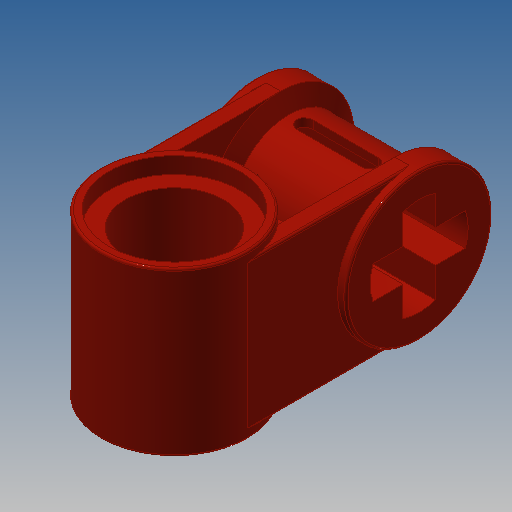
# Autodesk Inventor part: 6536-Red
Saved by Autodesk Inventor 2022.2 (Build 262287000, 287)
## iProperties
Created: 2014-07-19
Part Number: 6536-Red
Material: ABS Plastic
Document SubType Name: Modeling
Designer: D. Kohfeld
Mass: 0.381818 g
Surface Area: 7.9954 cm^2
Volume: 0.360206 cm^3
Density: 1.06 g/cm^3
Appearance: Red
Author: D. Kohfeld
Autodesk Inventor part; units mm, degrees
ref_plane "YZ Plane" through (0, 0, 0) normal (1, 0, 0) x (0, 1, 0)
ref_plane "XZ Plane" through (0, 0, 0) normal (0, 1, 0) x (-1, 0, 0)
sketch "Sketch2" plane through (0, 0, 0) normal (0, 1, 0) x (-1, 0, 0)
  circle A0 centre (0, 0) radius 3.6
  circle A1 centre (0, 0) radius 2.4
  line L0 (-3.6, -8) -> (3.6, -8)
  line L1 (-4, -8) -> (-4, -11.6)
  line L2 (-4, -11.6) -> (-2.8, -11.6)
  line L3 (-2.8, -11.6) -> (-2.4, -10.8)
  line L4 (-2.4, -10.8) -> (2.4, -10.8)
  line L5 (2.4, -10.8) -> (2.8, -11.6)
  line L6 (2.8, -11.6) -> (4, -11.6)
  line L7 (4, -11.6) -> (4, -8)
  line L8 (4, -8) -> (-4, -8)
  line L9 (3.6, -8) -> (3.6, 0)
  line L10 (-3.6, -8) -> (-3.6, 0)
  line L11 (-1.6, -7.6) -> (1.6, -7.6)
  arc A2 (1.6, -8.4) -> (1.6, -7.6) centre (1.6, -8) ccw
  line L12 (1.6, -8.4) -> (-1.6, -8.4)
  arc A3 (-1.6, -7.6) -> (-1.6, -8.4) centre (-1.6, -8) ccw
  point P0 (0, -8)
  point P1 (0, -7.6)
  dimension "d0" = 7.2
  dimension "d1" = 4.8
  dimension "d2" = 8
  dimension "d13" = 7.2
  dimension "d14" = 1.2
  dimension "d15" = 8
  dimension "d16" = 5.6
  dimension "d17" = 1.6
  dimension "d18" = 0.8
  dimension "d19" = 4
  constraints: 26 end point, 6 point on circle, 6 tangent, 4 centre point, 4 parallel, 3 equal length, 3 midpoint, 3 perpendicular, 2 coincident, 2 vertical, 1 collinear, 1 horizontal, 1 horizontal alignment, 1 vertical alignment
  measures "d0" diameter of A0
  measures "d1" diameter of A1
  measures "d2" distance from line of L0 A0.centre
  measures "d13" diameter of L2 L0
  measures "d14" distance from line of L2.end L1
  measures "d15" distance between parallel lines of L7 L1
  measures "d16" diameter of L4 L0
  measures "d17" distance from line of L3.end L1
  measures "d18" distance between parallel lines of L12 L11
sketch "Sketch2 outline for Extrusion1" plane through (0, 0, 0) normal (0, 1, 0) x (-1, 0, 0)
  circle A0 centre (0, 0) radius 3.6
  circle A1 centre (0, 0) radius 2.4
extrude "Extrusion1" add sketch "Sketch2 outline for Extrusion1" along normal mid plane 8
sketch "Sketch4" plane through (0, 4, 0) normal (0, 1, 0) x (1, 0, 0)
  circle A0 centre (0, 0) radius 2.4 projected
  circle A1 centre (0, 0) radius 3.6 projected
  circle A2 centre (0, 0) radius 3.2
  dimension "d10" = 6.4
  constraints: 1 centre point, 1 coincident
  measures "d10" diameter of A2
sketch "Sketch4 outline for Extrusion3" plane through (0, 4, 0) normal (0, 1, 0) x (1, 0, 0)
  circle A0 centre (0, 0) radius 3.2
  circle A1 centre (0, 0) radius 2.4
extrude "Extrusion3" cut sketch "Sketch4 outline for Extrusion3" against normal blind 0.8
mirror "Mirror1" about plane through (0, 0, 0) normal (0, 1, 0) of "Extrusion3"
ref_plane "Work Plane1" through (3.6, 0, -8) normal (0, 0, -1) x (-1, 0, 0)
sketch "Sketch3" plane through (3.6, 0, -8) normal (0, 0, -1) x (-1, 0, 0)
  line L0 (0, -4) -> (0, 4) projected
  line L1 (7.2, -4) -> (7.2, 4) projected
  line L2 (0, 3.6) -> (0.8, 3.6)
  line L3 (0.8, 3.6) -> (0.8, -3.6)
  line L4 (0.8, -3.6) -> (0, -3.6)
  line L5 (0, -3.6) -> (0, 3.6)
  line L6 (7.2, 3.6) -> (6.4, 3.6)
  line L7 (6.4, 3.6) -> (6.4, -3.6)
  line L8 (6.4, -3.6) -> (7.2, -3.6)
  line L9 (7.2, -3.6) -> (7.2, 3.6)
  point P0 (3.6, 0)
  point P1 (0, 0)
  point P2 (7.2, 0)
  dimension "d6" = 7.2
  dimension "d7" = 0.8
  constraints: 16 end point, 4 midpoint, 4 parallel, 2 equal length, 2 horizontal, 2 perpendicular, 2 point on line
  measures "d6" distance between parallel lines of L4 L2
  measures "d7" distance between parallel lines of L0 L3
sketch "Sketch3 outline for Extrusion2" plane through (3.6, 0, -8) normal (0, 0, -1) x (-1, 0, 0)
  line L0 (0.8, 3.6) -> (0, 3.6)
  line L1 (0, 3.6) -> (0, -3.6)
  line L2 (0, -3.6) -> (0.8, -3.6)
  line L3 (0.8, -3.6) -> (0.8, 3.6)
  line L4 (7.2, -3.6) -> (7.2, 3.6)
  line L5 (7.2, 3.6) -> (6.4, 3.6)
  line L6 (6.4, 3.6) -> (6.4, -3.6)
  line L7 (6.4, -3.6) -> (7.2, -3.6)
extrude "Extrusion2" add sketch "Sketch3 outline for Extrusion2" against normal up to next
sketch "Sketch2 outline for Revolution1" plane through (0, 0, 0) normal (0, 1, 0) x (-1, 0, 0)
  line L0 (-4, -11.6) -> (-4, -8)
  line L1 (-4, -8) -> (4, -8)
  line L2 (4, -8) -> (4, -11.6)
  line L3 (4, -11.6) -> (2.8, -11.6)
  line L4 (2.8, -11.6) -> (2.4, -10.8)
  line L5 (2.4, -10.8) -> (-2.4, -10.8)
  line L6 (-2.4, -10.8) -> (-2.8, -11.6)
  line L7 (-2.8, -11.6) -> (-4, -11.6)
revolve "Revolution1" add sketch "Sketch2 outline for Revolution1" angle 360 about axis through (-4, 0, -8) along (1, 0, 0)
sketch "Sketch2 outline for Extrusion4" plane through (0, 0, 0) normal (0, 1, 0) x (-1, 0, 0)
  line L0 (-3.6, 0) -> (-3.6, -8)
  arc A0 (3.6, 0) -> (-3.6, 0) centre (0, 0) cw
  line L1 (3.6, -8) -> (3.6, 0)
  line L2 (0, -8) -> (3.6, -8)
  line L3 (-3.6, -8) -> (0, -8)
extrude "Extrusion4" add sketch "Sketch2 outline for Extrusion4" along normal mid plane 1.6
sketch "Sketch2 outline for Extrusion5" plane through (0, 0, 0) normal (0, 1, 0) x (-1, 0, 0)
  line L0 (-1.6, -7.6) -> (1.6, -7.6)
  arc A0 (1.6, -7.6) -> (1.6, -8.4) centre (1.6, -8) cw
  line L1 (1.6, -8.4) -> (-1.6, -8.4)
  arc A1 (-1.6, -8.4) -> (-1.6, -7.6) centre (-1.6, -8) cw
extrude "Extrusion5" cut sketch "Sketch2 outline for Extrusion5" along normal through all both and the other way through all
sketch "Sketch5" plane through (4, 0, -8) normal (1, 0, 0) x (0, 0, -1)
  circle A0 centre (0, 0) radius 3.6
  circle A1 centre (0, 0) radius 2.4 construction
  line L0 (-0.8, 2.262742) -> (-0.8, 0.8)
  line L1 (-0.8, 0.8) -> (-2.262742, 0.8)
  line L2 (-2.262742, -0.8) -> (-0.8, -0.8)
  line L3 (-0.8, -0.8) -> (-0.8, -2.262742)
  line L4 (0.8, -2.262742) -> (0.8, -0.8)
  line L5 (0.8, -0.8) -> (2.262742, -0.8)
  line L6 (2.262742, 0.8) -> (0.8, 0.8)
  line L7 (0.8, 0.8) -> (0.8, 2.262742)
  arc A2 (0.8, 2.262742) -> (-0.8, 2.262742) centre (0, 0) ccw
  arc A3 (-2.262742, 0.8) -> (-2.262742, -0.8) centre (0, 0) ccw
  arc A4 (-0.8, -2.262742) -> (0.8, -2.262742) centre (0, 0) ccw
  arc A5 (2.262742, -0.8) -> (2.262742, 0.8) centre (0, 0) ccw
  point P0 (-8, 0)
  dimension "d25" = 4.8
  dimension "d26" = 1.6
  constraints: 16 end point, 8 point on circle, 7 equal length, 4 centre point, 4 perpendicular, 3 parallel, 1 coincident, 1 vertical, 14 other
  measures "d26" distance between parallel lines of L7 L0
sketch "Sketch5 outline for Extrusion6" plane through (4, 0, -8) normal (1, 0, 0) x (0, 0, -1)
  arc A0 (0.8, 2.262742) -> (-0.8, 2.262742) centre (0, 0) ccw
  line L0 (0.8, 0.8) -> (0.8, 2.262742)
  line L1 (2.262742, 0.8) -> (0.8, 0.8)
  arc A1 (2.262742, -0.8) -> (2.262742, 0.8) centre (0, 0) ccw
  line L2 (0.8, -0.8) -> (2.262742, -0.8)
  line L3 (0.8, -2.262742) -> (0.8, -0.8)
  arc A2 (-0.8, -2.262742) -> (0.8, -2.262742) centre (0, 0) ccw
  line L4 (-0.8, -0.8) -> (-0.8, -2.262742)
  line L5 (-2.262742, -0.8) -> (-0.8, -0.8)
  arc A3 (-2.262742, 0.8) -> (-2.262742, -0.8) centre (0, 0) ccw
  line L6 (-0.8, 0.8) -> (-2.262742, 0.8)
  line L7 (-0.8, 2.262742) -> (-0.8, 0.8)
extrude "Extrusion6" cut sketch "Sketch5 outline for Extrusion6" against normal through all
fillet "Fillet1" radius 0.1 8 edges at (3.6, 4, 0) (3.6, -4, 0) (3.6, 3.6, -4) (-3.6, 3.6, -4) (-4, 0, -4.4) (3.6, -3.6, -4) (-3.6, -3.6, -4) (4, 0, -4.4)
equation "\"d0\" = tlad"
equation "\"d1\" = tpd"
equation "\"d2\" = lu"
equation "\"d13\" = tlad"
equation "\"d15\" = lu"
equation "\"d17\" = wall"
equation "\"d10\" = tsd"
equation "\"d11\" = tsl"
equation "\"d6\" = tlad"
equation "\"d7\" = tsl"
equation "\"d21\" = wall"
equation "\"d25\" = kd"
equation "\"d26\" = axlet"
equation "\"tlad\" = 7.2"
equation "\"tpd\" = 4.8"
equation "\"lu\" = 8"
equation "\"wall\" = 1.6"
equation "\"tsd\" = 6.4"
equation "\"tsl\" = 0.8"
equation "\"kd\" = 4.8"
equation "\"axlet\" = 1.6"
body "Solid1"
